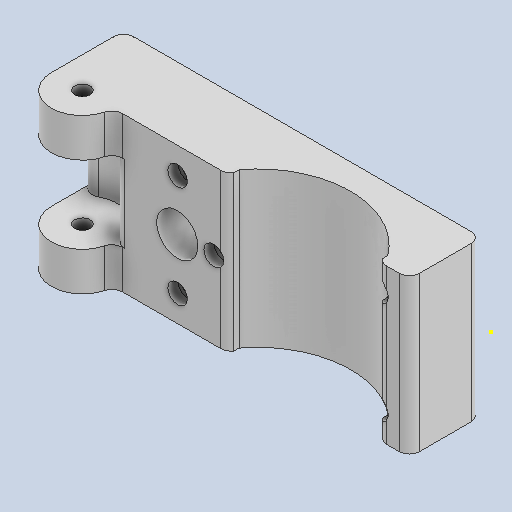
# Autodesk Inventor part: Bike_Mount_Right_v2
Saved by Autodesk Inventor 2023.1 (Build 271208000, 208)
## iProperties
Created: 2023-01-23
Part Number: Bike_Mount_Right_v2
Material: Generic
Document SubType Name: Modeling
Designer: manny
Density: 1 g/cm^3
Appearance: Default
Author: manny
Autodesk Inventor part; units mm, degrees
ref_plane "YZ Plane" through (0, 0, 0) normal (1, 0, 0) x (0, 1, 0)
ref_plane "XZ Plane" through (0, 0, 0) normal (0, 1, 0) x (-1, 0, 0)
ref_plane "XY Plane" through (0, 0, 0) normal (0, 0, 1) x (1, 0, 0)
sketch "Sketch2" plane through (0, 0, 0) normal (0, 1, 0) x (-1, 0, 0)
  line L0 (3.9324, 0) -> (5, 0)
  arc A0 (3.9324, 0) -> (1.9324, -2) centre (3.9324, -2) ccw
  line L1 (3.9324, 0) -> (6.9065, 0)
  line L2 (3.9324, 0) -> (6.3389, 0)
  arc A1 (7.9907, -0.8725) -> (36.874, -0.8725) centre (22.4324, 8.9853) ccw
  line L3 (38.5258, 0) -> (57.6864, 0)
  arc A2 (71.4324, 0) -> (59.6229, 1.5) centre (65.4324, 0) ccw
  circle A3 centre (65.4324, 0) radius 1.5
  arc A4 (57.6864, 0) -> (59.6229, 1.5) centre (57.6864, 2) ccw
  arc A5 (38.5258, 0) -> (36.874, -0.8725) centre (38.5258, -2) ccw
  arc A6 (7.9907, -0.8725) -> (6.3389, 0) centre (6.3389, -2) ccw
  arc A7 (59.3504, -1.7983) -> (57.1879, 0) centre (57.1879, -2.1995) ccw
  line L4 (77.1831, 8.9853) -> (-10.6505, 8.9853) construction
  line L5 (3.9324, 17.9706) -> (5, 17.9706)
  arc A8 (42.998, 40.9699) -> (1.9324, 19.9706) centre (55.0831, -33.3161) ccw
  arc A9 (1.9324, 19.9706) -> (3.9324, 17.9706) centre (3.9324, 19.9706) ccw
  line L6 (3.9324, 17.9706) -> (6.9065, 17.9706)
  line L7 (3.9324, 17.9706) -> (6.3389, 17.9706)
  arc A10 (36.874, 18.843) -> (7.9907, 18.843) centre (22.4324, 8.9853) ccw
  line L8 (38.5258, 17.9706) -> (57.6864, 17.9706)
  arc A11 (59.6229, 16.4706) -> (71.4324, 17.9706) centre (65.4324, 17.9706) ccw
  arc A12 (71.4324, 17.9706) -> (42.998, 40.9699) centre (43.4479, 12.4496) ccw
  circle A13 centre (65.4324, 17.9706) radius 1.5
  arc A14 (59.6229, 16.4706) -> (57.6864, 17.9706) centre (57.6864, 15.9706) ccw
  arc A15 (36.874, 18.843) -> (38.5258, 17.9706) centre (38.5258, 19.9706) ccw
  arc A16 (6.3389, 17.9706) -> (7.9907, 18.843) centre (6.3389, 19.9706) ccw
  arc A17 (65.6797, 24.421) -> (59.3504, 19.7689) centre (64.5387, 19.3419) ccw
  arc A18 (65.6797, 24.421) -> (67.6049, 27.617) centre (65.5936, 26.6507) ccw
  arc A19 (57.1879, 17.9706) -> (59.3504, 19.7689) centre (57.1879, 20.1701) ccw
  line L9 (1.9324, -2) -> (1.9324, -12)
  line L10 (3.9324, -14) -> (69.4324, -14)
  arc A20 (1.9324, -12) -> (3.9324, -14) centre (3.9324, -12) ccw
  line L11 (71.4324, 0) -> (71.4324, -12)
  arc A21 (69.4324, -14) -> (71.4324, -12) centre (69.4324, -12) ccw
  arc A22 (59.3504, -1.7983) -> (71.4324, -2.4583) centre (65.4715, -0.6626) ccw
  point P0 (0, 0)
  point P1 (7.4324, 0)
  point P2 (37.4324, 0)
  point P3 (22.4324, -8.5)
  point P4 (0, 17.9706)
  point P5 (7.4324, 17.9706)
  point P6 (37.4324, 17.9706)
  point P7 (22.4324, 26.4706)
  point P8 (71.4324, 17.9706)
  point P9 (6.3389, 17.9706)
  dimension "d3" = 2
  dimension "d12" = 3.5
  dimension "d13" = 30
  dimension "d14" = 8.5
  dimension "d17" = 3
  dimension "d18" = 2
  dimension "d19" = 2
  dimension "d21" = 0
  dimension "d22" = 0
  dimension "d91" = 3.9324
  dimension "d92" = 2
  dimension "d93" = 28
  dimension "d94" = 2
  dimension "d107" = 10
  constraints: 51 point on circle, 25 symmetric about line, 24 end point, 23 centre point, 15 tangent, 11 point on line, 5 horizontal, 2 coincident, 2 vertical, 1 equal radius, 8 other
  measures "d3" radius of A0
  measures "d12" distance of L0.start point (7.432, 0)
  measures "d13" distance of point (7.432, 0) point (37.432, 0)
  measures "d14" vertical distance of point (7.432, 0) point (22.432, -8.5)
  measures "d17" diameter of A3
  measures "d18" radius of A4
  measures "d19" radius of A6
  measures "d21" vertical distance of point (0, 0) A2.centre
  measures "d22" distance from line of point (0, 0) L3
  measures "d91" distance of L0.start point (0, 0)
  measures "d92" radius of A20
  measures "d93" distance of A2.centre point (37.432, 0)
  measures "d94" radius of A21
  measures "d107" distance of L9.start L9.end
extrude "Extrusion1" add sketch "Sketch2" along normal mid plane 30 contours L0 L1 A6 A1 A5 L3 A7 A22 L11 A21 L10 A20 L9 A0 | L3 A4 A2 L11 A22 A7
extrude "Extrusion2" cut sketch "Sketch2" along normal mid plane 15 contours L3 A4 A2 L11 A22 A7
sketch "Sketch7" plane through (0, -15, 0) normal (0, -1, 0) x (1, 0, 0)
  arc A0 (-6.3389, 0) -> (-7.9907, -0.8725) centre (-6.3389, -2) ccw projected
  line L0 (-7.9907, -0.8725) -> (-7.9907, -1.8725)
  arc A1 (-36.874, -0.8725) -> (-7.9907, -0.8725) centre (-22.4324, 8.9853) ccw projected
  line L1 (-36.874, -0.8725) -> (-36.874, -1.8725)
  arc A2 (-36.874, -1.8725) -> (-7.9907, -1.8725) centre (-22.4324, 8.9853) ccw
  point P0 (0, 0)
  dimension "d59" = 1
  dimension "d60" = 1
  constraints: 4 end point, 2 point on circle, 2 vertical, 1 centre point
  measures "d59" distance of L0.start L0.end
  measures "d60" distance of L1.start L1.end
extrude "Extrusion10" cut sketch "Sketch7" against normal up to next
fillet "Fillet4" radius 2 1 edges at (-71.4324, 0, -2.4583)
sketch "Sketch13" plane through (-57.6864, -15, 0) normal (0, 0, 1) x (1, 0, 0)
  circle A0 centre (10.6864, 15) radius 4
  line L0 (55.754, 30) -> (55.754, 0) projected
  point P0 (57.6864, 15)
  dimension "d99" = 8
  dimension "d106" = 47
  constraints: 1 centre point
  measures "d99" diameter of A0
  measures "d106" distance of A0.centre point (57.686, 15)
extrude "Extrusion15" cut sketch "Sketch13" against normal up to next
sketch "Sketch14" plane through (-3.9324, 15, -14) normal (0, 0, -1) x (-1, 0, 0)
  circle A0 centre (43.0676, -15) radius 4 projected
  line L0 (43.0676, -21.3509) -> (37.5676, -18.1754)
  line L1 (37.5676, -18.1754) -> (37.5676, -11.8246)
  line L2 (37.5676, -11.8246) -> (43.0676, -8.6491)
  line L3 (43.0676, -8.6491) -> (48.5676, -11.8246)
  line L4 (48.5676, -11.8246) -> (48.5676, -18.1754)
  line L5 (48.5676, -18.1754) -> (43.0676, -21.3509)
  line L6 (67.5, -30) -> (67.5, 0) projected
  point P0 (-3.9324, -15)
  point P1 (37.5676, -15)
  dimension "d103" = 11
  constraints: 12 end point, 1 coincident, 1 midpoint, 1 parallel, 13 other
  measures "d103" distance from line of point (37.568, -15) L4
extrude "Extrusion16" cut sketch "Sketch14" against normal blind 6
sketch "Sketch32" plane through (-3.9324, 15, -14) normal (0, 0, -1) x (-1, 0, 0)
  point P0 (-3.9324, -15)
sketch "Sketch33" plane through (-3.9324, 15, -14) normal (0, 0, -1) x (-1, 0, 0)
  point P0 (-3.9324, -15)
sketch "Sketch41" plane through (-3.9324, 15, -14) normal (0, 0, -1) x (-1, 0, 0)
  circle A0 centre (4, -5.1) radius 1.1
  circle A1 centre (4, -24.9) radius 1.1
  circle A2 centre (43, -5.1) radius 1.1
  circle A3 centre (43, -24.9) radius 1.1
  circle A4 centre (5.5, -15) radius 1.1
  circle A5 centre (36, -15) radius 1.1
  line L0 (0, 0) -> (65.5, 0) projected
  line L1 (-2, -30) -> (-2, 0) projected
  point P0 (-3.9324, -15)
  dimension "d254" = 2.2
  dimension "d255" = 19.8
  dimension "d256" = 39
  dimension "d257" = 5.1
  dimension "d258" = 6
  dimension "d259" = 9.9
  dimension "d260" = 30.5
  dimension "d261" = 1.5
  constraints: 6 centre point, 5 equal radius, 3 horizontal alignment, 2 vertical alignment
  measures "d254" diameter of A0
  measures "d255" distance of A1.centre A0.centre
  measures "d256" distance of A2.centre A0.centre
  measures "d257" distance from line of L0 A0.centre
  measures "d258" distance from line of L1 A0.centre
  measures "d259" vertical distance of A4.centre A0.centre
  measures "d260" distance of A5.centre A4.centre
  measures "d261" horizontal distance of A4.centre A0.centre
extrude "Extrusion36" cut sketch "Sketch41" against normal blind 20
sketch "Sketch42" plane through (-57.6864, -15, 0) normal (0, 0, 1) x (1, 0, 0)
  circle A0 centre (10.754, 24.9) radius 1.1 projected
  circle A1 centre (10.754, 24.9) radius 1.9
  circle A2 centre (17.754, 15) radius 1.1 projected
  circle A3 centre (17.754, 15) radius 1.9
  circle A4 centre (10.754, 5.1) radius 1.1 projected
  circle A5 centre (10.754, 5.1) radius 1.9
  circle A6 centre (49.754, 5.1) radius 1.1 projected
  circle A7 centre (49.754, 5.1) radius 1.9
  circle A8 centre (48.254, 15) radius 1.1 projected
  circle A9 centre (48.254, 15) radius 1.9
  circle A10 centre (49.754, 24.9) radius 1.1 projected
  circle A11 centre (49.754, 24.9) radius 1.9
  point P0 (57.6864, 15)
  dimension "d264" = 3.8
  constraints: 6 centre point, 6 coincident, 5 equal radius
  measures "d264" diameter of A1
extrude "Extrusion37" cut sketch "Sketch42" against normal blind 2 contours A0 | A1 | A2 | A3 | A4 | A5
extrude "Extrusion38" cut sketch "Sketch42" against normal blind 7.25 contours A10 | A11
extrude "Extrusion39" cut sketch "Sketch42" against normal blind 7.25 contours A8 | A9
extrude "Extrusion40" cut sketch "Sketch42" against normal blind 7.25 contours A6 | A7
body "Solid1"
